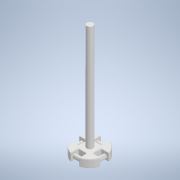
# Autodesk Inventor part: G-3
Saved by Autodesk Inventor 2022 (Build 260153000, 153)
## iProperties
Created: 2021-06-28
Part Number: G-3
Material: Generic
Document SubType Name: Modeling
Designer: Ranjita
Density: 1 g/cm^3
Appearance: Default
Author: Ranjita
Autodesk Inventor part; units mm, degrees
ref_plane "YZ Plane" through (0, 0, 0) normal (1, 0, 0) x (0, 1, 0)
ref_plane "XZ Plane" through (0, 0, 0) normal (0, 1, 0) x (-1, 0, 0)
ref_plane "XY Plane" through (0, 0, 0) normal (0, 0, 1) x (1, 0, 0)
sketch "Sketch1" plane through (0, 0, 0) normal (0, 1, 0) x (-1, 0, 0)
  arc A0 (1.665, -6.4537) -> (-1.665, -6.4537) centre (0, 0) ccw
  line L0 (0, 6.665) -> (0, 0)
  line L1 (0, -6.665) -> (0, 0) construction
  line L2 (-1.665, -6.4537) -> (-1.665, -3.1237)
  line L3 (-1.665, -3.1237) -> (1.665, -3.1237)
  line L4 (1.665, -3.1237) -> (1.665, -6.4537)
  line L5 (1.665, -6.4537) -> (-1.665, -3.1237) construction
  line L6 (-1.665, -6.4537) -> (1.665, -3.1237) construction
  line L7 (6.4537, -1.665) -> (3.1237, -1.665)
  line L8 (3.1237, -1.665) -> (3.1237, 1.665)
  line L9 (3.1237, 1.665) -> (6.4537, 1.665)
  line L10 (6.4537, 1.665) -> (3.1237, -1.665) construction
  line L11 (6.4537, -1.665) -> (3.1237, 1.665) construction
  line L12 (1.665, 6.4537) -> (1.665, 3.1237)
  line L13 (1.665, 3.1237) -> (-1.665, 3.1237)
  line L14 (-1.665, 3.1237) -> (-1.665, 6.4537)
  line L15 (-1.665, 6.4537) -> (1.665, 3.1237) construction
  line L16 (1.665, 6.4537) -> (-1.665, 3.1237) construction
  line L17 (-6.4537, 1.665) -> (-3.1237, 1.665)
  line L18 (-3.1237, 1.665) -> (-3.1237, -1.665)
  line L19 (-3.1237, -1.665) -> (-6.4537, -1.665)
  line L20 (-6.4537, -1.665) -> (-3.1237, 1.665) construction
  line L21 (-6.4537, 1.665) -> (-3.1237, -1.665) construction
  point P0 (0, -4.7887)
  point P1 (6.665, 0)
  point P2 (4.7887, 0)
  point P3 (0, 6.665)
  point P4 (0, 4.7887)
  point P5 (-6.665, 0)
  point P6 (-4.7887, 0)
  dimension "d0" = 13.33
  dimension "d1" = 3.33
  dimension "d4" = 360
  constraints: 44 end point, 8 midpoint, 3 point on circle, 2 vertical, 1 centre point, 1 coincident, 1 parallel, 1 perpendicular, 1 point on line, 45 other
  measures "d0" diameter of A0
  measures "d1" distance of L4.end L3.end
extrude "Extrusion1" add sketch "Sketch1" along normal blind 3.332 contours L4 L3 L2 A0 L19 L18 L17 L14 L13 L12 L9 L8 L7
sketch "Sketch2" plane through (1.665, 0, -6.4537) normal (-1, 0, 0) x (0, 0, 1)
  line L0 (3.33, 0) -> (3.33, 3.332) construction
  line L1 (3.33, 1.4886) -> (-0.0199, 1.4886) construction
  circle A0 centre (1.655, 1.4886) radius 0.83
  point P0 (6.4537, 0)
  dimension "d8" = 1.66
  constraints: 2 end point, 1 centre point, 1 horizontal, 1 midpoint, 1 point on line
  measures "d8" diameter of A0
extrude "Extrusion2" add sketch "Sketch2" along normal blind 3.332
pattern_circular "Circular Pattern1" count 4 over 360 about axis through (0, 0, 0) along (0, 1, 0) of "Extrusion2"
sketch "Sketch3" plane through (0, 3.332, 0) normal (0, 1, 0) x (1, 0, 0)
  circle A0 centre (0, 0) radius 1.33
  dimension "d14" = 2.66
  constraints: 1 centre point, 1 coincident
  measures "d14" diameter of A0
extrude "Extrusion3" add sketch "Sketch3" along normal blind 30
fillet "Fillet1" radius 0.3 49 edges at (-4.7129, 0, -4.7129) (-1.665, 0, -4.7887) (0, 0, -3.1237) (1.665, 0, -4.7887) (4.7129, 0, -4.7129) (4.7887, 0, -1.665) (3.1237, 0, 0) (4.7887, 0, 1.665) (4.7129, 0, 4.7129) (1.665, 0, 4.7887) (0, 0, 3.1237) (-1.665, 0, 4.7887) (-4.7129, 0, 4.7129) (-4.7887, 0, 1.665) (-3.1237, 0, 0) (-4.7887, 0, -1.665) (-4.7129, 3.332, -4.7129) (-4.7887, 3.332, -1.665) (-3.1237, 3.332, 0) (-4.7887, 3.332, 1.665) (-4.7129, 3.332, 4.7129) (-1.665, 3.332, 4.7887) (0, 3.332, 3.1237) (1.665, 3.332, 4.7887) (4.7129, 3.332, 4.7129) (4.7887, 3.332, 1.665) (3.1237, 3.332, 0) (4.7887, 3.332, -1.665) (4.7129, 3.332, -4.7129) (1.665, 3.332, -4.7887) (0, 3.332, -3.1237) (-1.665, 3.332, -4.7887) (1.665, 1.4886, 5.6286) (-1.665, 1.666, 6.4537) (-6.4537, 1.666, 1.665) (-3.1237, 1.666, -1.665) (-6.4537, 1.666, -1.665) (-3.1237, 1.666, 1.665) (-1.665, 1.666, -3.1237) (1.665, 1.666, -3.1237) (-1.665, 1.4886, -5.6286) (1.665, 1.666, -6.4537) (6.4537, 1.666, -1.665) (3.1237, 1.666, -1.665) (3.1237, 1.666, 1.665) (6.4537, 1.666, 1.665) (1.665, 1.666, 6.4537) (1.665, 1.666, 3.1237) (-1.665, 1.666, 3.1237)
sketch "Sketch4" plane through (0, 33.332, 0) normal (0, 1, 0) x (1, 0, 0)
  circle A0 centre (0, 0) radius 1.33
  constraints: 1 centre point, 1 coincident
extrude "Extrusion4" add sketch "Sketch4" along normal blind 15
body "Solid1"
